Autodesk Inventor part; units mm, degrees
(part 2 of 2)
  spline S326 degree 2 poles (59.0858, 25.3317) (58.8361, 25.3317) (58.5495, 25.5905) (58.5495, 25.8217) knots 0 0 0 1 2 2 2
  spline S327 degree 2 poles (58.5495, 25.8217) (58.5495, 26.0482) (58.887, 26.3209) (59.1921, 26.3209) knots 0 0 0 1 2 2 2
  line L134 (59.1921, 26.3209) -> (59.3539, 26.3209)
  line L135 (65.4232, 23.2885) -> (65.4232, 23.307)
  spline S328 degree 2 poles (65.4232, 23.307) (65.3492, 23.0851) (64.9101, 22.7616) (64.397, 22.5952) (64.0919, 22.5952) knots 0 0 0 1 2 3 3 3
  spline S329 degree 2 poles (64.0919, 22.5952) (63.6851, 22.5952) (63.001, 22.9372) (62.5018, 23.5659) (62.2475, 24.4026) (62.2475, 24.8925) knots 0 0 0 1 2 3 4 4 4
  spline S330 degree 2 poles (62.2475, 24.8925) (62.2475, 25.9234) (63.2691, 27.0929) (64.1104, 27.0929) knots 0 0 0 1 2 2 2
  spline S331 degree 2 poles (64.1104, 27.0929) (64.5911, 27.0929) (65.2568, 26.76) (65.4232, 26.4503) knots 0 0 0 1 2 2 2
  line L136 (65.4232, 26.4503) -> (65.4232, 27.948)
  spline S332 degree 2 poles (65.4232, 27.948) (65.4232, 28.3039) (65.7283, 28.6922) (66.0149, 28.6922) knots 0 0 0 1 2 2 2
  spline S333 degree 2 poles (66.0149, 28.6922) (66.2922, 28.6922) (66.6019, 28.3317) (66.6019, 28.0035) knots 0 0 0 1 2 2 2
  line L137 (66.6019, 28.0035) -> (66.6019, 23.2885)
  spline S334 degree 2 poles (66.6019, 23.2885) (66.6019, 22.9511) (66.2737, 22.5952) (66.0149, 22.5952) knots 0 0 0 1 2 2 2
  spline S335 degree 2 poles (66.0149, 22.5952) (65.756, 22.5952) (65.4232, 22.9603) (65.4232, 23.2885) knots 0 0 0 1 2 2 2
  spline S336 degree 2 poles (63.4864, 24.8556) (63.4864, 24.4349) (63.7406, 23.8617) (64.1705, 23.5798) (64.4201, 23.5798) knots 0 0 0 1 2 3 3 3
  spline S337 degree 2 poles (64.4201, 23.5798) (64.679, 23.5798) (65.1042, 23.8479) (65.3631, 24.421) (65.3631, 24.8556) knots 0 0 0 1 2 3 3 3
  spline S338 degree 2 poles (65.3631, 24.8556) (65.3631, 25.2623) (65.1042, 25.8448) (64.6697, 26.1406) (64.4155, 26.1406) knots 0 0 0 1 2 3 3 3
  spline S339 degree 2 poles (64.4155, 26.1406) (64.1474, 26.1406) (63.7267, 25.8355) (63.4864, 25.2531) (63.4864, 24.8556) knots 0 0 0 1 2 3 3 3
  spline S340 degree 2 poles (68.4047, 22.5952) (68.1274, 22.5952) (67.7252, 22.9557) (67.7252, 23.2747) knots 0 0 0 1 2 2 2
  spline S341 degree 2 poles (67.7252, 23.2747) (67.7252, 23.5428) (68.1089, 23.9357) (68.3908, 23.9357) knots 0 0 0 1 2 2 2
  spline S342 degree 2 poles (68.3908, 23.9357) (68.6728, 23.9357) (69.0703, 23.5474) (69.0703, 23.2747) knots 0 0 0 1 2 2 2
  spline S343 degree 2 poles (69.0703, 23.2747) (69.0703, 22.9603) (68.6728, 22.5952) (68.4047, 22.5952) knots 0 0 0 1 2 2 2
  line L138 (71.3169, 26.4365) -> (71.3169, 26.3902)
  spline S344 degree 2 poles (71.3169, 26.3902) (71.4556, 26.7369) (72.1628, 27.1021) (72.6204, 27.1021) knots 0 0 0 1 2 2 2
  spline S345 degree 2 poles (72.6204, 27.1021) (73.0642, 27.1021) (73.7714, 26.7138) (73.9471, 26.3579) knots 0 0 0 1 2 2 2
  spline S346 degree 2 poles (73.9471, 26.3579) (74.058, 26.1499) (74.1227, 25.6737) (74.1227, 25.3178) knots 0 0 0 1 2 2 2
  line L139 (74.1227, 25.3178) -> (74.1227, 23.3301)
  spline S347 degree 2 poles (74.1227, 23.3301) (74.1227, 22.9742) (73.7853, 22.5952) (73.5126, 22.5952) knots 0 0 0 1 2 2 2
  spline S348 degree 2 poles (73.5126, 22.5952) (73.2352, 22.5952) (72.8932, 22.9835) (72.8932, 23.3301) knots 0 0 0 1 2 2 2
  line L140 (72.8932, 23.3301) -> (72.8932, 25.1098)
  spline S349 degree 2 poles (72.8932, 25.1098) (72.8932, 25.6183) (72.6297, 26.1175) (72.2414, 26.1175) knots 0 0 0 1 2 2 2
  spline S350 degree 2 poles (72.2414, 26.1175) (71.9825, 26.1175) (71.5572, 25.8078) (71.4417, 25.4981) knots 0 0 0 1 2 2 2
  spline S351 degree 2 poles (71.4417, 25.4981) (71.3816, 25.3132) (71.3816, 24.6707) knots 0 0 0 1 1 1
  line L141 (71.3816, 24.6707) -> (71.3816, 23.3301)
  spline S352 degree 2 poles (71.3816, 23.3301) (71.3816, 22.9696) (71.0349, 22.5952) (70.7576, 22.5952) knots 0 0 0 1 2 2 2
  spline S353 degree 2 poles (70.7576, 22.5952) (70.4895, 22.5952) (70.1474, 22.9835) (70.1474, 23.3301) knots 0 0 0 1 2 2 2
  line L142 (70.1474, 23.3301) -> (70.1474, 26.418)
  spline S354 degree 2 poles (70.1474, 26.418) (70.1474, 26.7508) (70.4571, 27.1021) (70.7252, 27.1021) knots 0 0 0 1 2 2 2
  spline S355 degree 2 poles (70.7252, 27.1021) (70.8916, 27.1021) (71.1597, 26.9449) (71.3169, 26.6398) (71.3169, 26.4365) knots 0 0 0 1 2 3 3 3
  line L143 (75.1258, 23.3301) -> (75.1258, 27.9619)
  spline S356 degree 2 poles (75.1258, 27.9619) (75.1258, 28.3132) (75.454, 28.6922) (75.736, 28.6922) knots 0 0 0 1 2 2 2
  spline S357 degree 2 poles (75.736, 28.6922) (76.018, 28.6922) (76.36, 28.3178) (76.36, 27.9619) knots 0 0 0 1 2 2 2
  line L144 (76.36, 27.9619) -> (76.36, 23.3301)
  spline S358 degree 2 poles (76.36, 23.3301) (76.36, 22.9696) (76.0133, 22.5952) (75.736, 22.5952) knots 0 0 0 1 2 2 2
  spline S359 degree 2 poles (75.736, 22.5952) (75.4633, 22.5952) (75.1258, 22.9835) (75.1258, 23.3301) knots 0 0 0 1 2 2 2
  line L145 (8.8947, 4.4889) -> (7.716, 4.4889)
  line L146 (7.716, 4.4889) -> (7.716, 5.9819)
  line L147 (7.716, 5.9819) -> (6.2183, 5.9819)
  line L148 (6.2183, 5.9819) -> (6.2183, 7.1699)
  line L149 (6.2183, 7.1699) -> (7.716, 7.1699)
  line L150 (7.716, 7.1699) -> (7.716, 8.6676)
  line L151 (7.716, 8.6676) -> (8.8947, 8.6676)
  line L152 (8.8947, 8.6676) -> (8.8947, 7.1699)
  line L153 (8.8947, 7.1699) -> (10.4016, 7.1699)
  line L154 (10.4016, 7.1699) -> (10.4016, 5.9819)
  line L155 (10.4016, 5.9819) -> (8.8947, 5.9819)
  line L156 (8.8947, 5.9819) -> (8.8947, 4.4889)
  spline S360 degree 2 poles (12.944, 7.2901) (13.2722, 7.2901) (13.7437, 7.6692) (13.7437, 8.0297) knots 0 0 0 1 2 2 2
  spline S361 degree 2 poles (13.7437, 8.0297) (13.7437, 8.2932) (13.3739, 8.6815) (13.0596, 8.6815) knots 0 0 0 1 2 2 2
  spline S362 degree 2 poles (13.0596, 8.6815) (12.8377, 8.6815) (12.5603, 8.5613) (12.4032, 8.3718) (12.2275, 7.9927) (12.1767, 7.8818) knots 0 0 0 1 2 3 4 4 4
  spline S363 degree 2 poles (12.1767, 7.8818) (12.1258, 7.7662) (11.8808, 7.6553) (11.7283, 7.6553) knots 0 0 0 1 2 2 2
  spline S364 degree 2 poles (11.7283, 7.6553) (11.5341, 7.6553) (11.2244, 7.9604) (11.2244, 8.2054) knots 0 0 0 1 2 2 2
  spline S365 degree 2 poles (11.2244, 8.2054) (11.2244, 8.4319) (11.4879, 8.908) (11.9871, 9.3333) (12.7175, 9.5921) (13.1659, 9.5921) knots 0 0 0 1 2 3 4 4 4
  spline S366 degree 2 poles (13.1659, 9.5921) (13.5588, 9.5921) (14.2152, 9.3749) (14.7052, 8.9588) (14.9548, 8.4134) (14.9548, 8.099) knots 0 0 0 1 2 3 4 4 4
  spline S367 degree 2 poles (14.9548, 8.099) (14.9548, 7.6876) (14.5942, 7.0913) (14.2984, 6.8926) knots 0 0 0 1 2 2 2
  spline S368 degree 2 poles (14.2984, 6.8926) (14.5711, 6.7816) (15.0103, 6.3379) (15.2321, 5.797) (15.2321, 5.4827) knots 0 0 0 1 2 3 3 3
  spline S369 degree 2 poles (15.2321, 5.4827) (15.2321, 5.1129) (14.9317, 4.4149) (14.3539, 3.8695) (13.5588, 3.5644) (13.0827, 3.5644) knots 0 0 0 1 2 3 4 4 4
  spline S370 degree 2 poles (13.0827, 3.5644) (12.5927, 3.5644) (11.8161, 3.9157) (11.3169, 4.4427) (11.058, 5.0112) (11.058, 5.2054) knots 0 0 0 1 2 3 4 4 4
  spline S371 degree 2 poles (11.058, 5.2054) (11.058, 5.4688) (11.4001, 5.7924) (11.6543, 5.7924) knots 0 0 0 1 2 2 2
  spline S372 degree 2 poles (11.6543, 5.7924) (11.7884, 5.7924) (12.0334, 5.6306) (12.0796, 5.4873) knots 0 0 0 1 2 2 2
  spline S373 degree 2 poles (12.0796, 5.4873) (12.2737, 4.9881) (12.7036, 4.4981) (13.0919, 4.4981) knots 0 0 0 1 2 2 2
  spline S374 degree 2 poles (13.0919, 4.4981) (13.3138, 4.4981) (13.7206, 4.7154) (13.9933, 5.1499) (13.9933, 5.4365) knots 0 0 0 1 2 3 3 3
  spline S375 degree 2 poles (13.9933, 5.4365) (13.9933, 5.8618) (13.5357, 6.3333) (13.1289, 6.3333) knots 0 0 0 1 2 2 2
  spline S376 degree 2 poles (13.1289, 6.3333) (13.0596, 6.3333) (12.7314, 6.3009) (12.6759, 6.3009) knots 0 0 0 1 2 2 2
  spline S377 degree 2 poles (12.6759, 6.3009) (12.4263, 6.3009) (12.1397, 6.5598) (12.1397, 6.7909) knots 0 0 0 1 2 2 2
  spline S378 degree 2 poles (12.1397, 6.7909) (12.1397, 7.0174) (12.4771, 7.2901) (12.7822, 7.2901) knots 0 0 0 1 2 2 2
  line L157 (12.7822, 7.2901) -> (12.944, 7.2901)
  line L158 (17.7976, 4.2809) -> (17.7976, 7.7616)
  spline S379 degree 2 poles (17.7976, 7.7616) (16.9147, 6.9989) (16.5403, 6.9989) knots 0 0 0 1 1 1
  spline S380 degree 2 poles (16.5403, 6.9989) (16.3415, 6.9989) (16.0411, 7.3086) (16.0411, 7.5166) knots 0 0 0 1 2 2 2
  spline S381 degree 2 poles (16.0411, 7.5166) (16.0411, 7.757) (16.323, 7.9696) (16.6559, 8.1222) knots 0 0 0 1 2 2 2
  spline S382 degree 2 poles (16.6559, 8.1222) (17.1135, 8.3394) (17.6636, 8.8202) (18.0981, 9.4211) (18.2645, 9.6014) (18.4864, 9.6014) knots 0 0 0 1 2 3 4 4 4
  spline S383 degree 2 poles (18.4864, 9.6014) (18.736, 9.6014) (19.0272, 9.2269) (19.0272, 8.9219) knots 0 0 0 1 2 2 2
  line L159 (19.0272, 8.9219) -> (19.0272, 4.4334)
  spline S384 degree 2 poles (19.0272, 4.4334) (19.0272, 3.5644) (18.4078, 3.5644) knots 0 0 0 1 1 1
  spline S385 degree 2 poles (18.4078, 3.5644) (18.1304, 3.5644) (17.7976, 3.9342) (17.7976, 4.2809) knots 0 0 0 1 2 2 2
  spline S386 degree 2 poles (20.9039, 5.8202) (20.9039, 6.4211) (21.1119, 7.4658) (21.528, 8.4688) (21.8423, 8.9819) knots 0 0 0 1 2 3 3 3
  spline S387 degree 2 poles (21.8423, 8.9819) (22.0272, 9.2917) (22.2999, 9.5829) (22.5588, 9.6615) (22.7483, 9.6615) knots 0 0 0 1 2 3 3 3
  spline S388 degree 2 poles (22.7483, 9.6615) (23.021, 9.6615) (23.021, 9.4766) knots 0 0 0 1 1 1
  spline S389 degree 2 poles (23.021, 9.4766) (23.021, 9.4257) (22.6512, 8.6214) (22.3415, 7.7893) (22.0734, 6.5274) (22.0734, 5.8202) knots 0 0 0 1 2 3 4 4 4
  spline S390 degree 2 poles (22.0734, 5.8202) (22.0734, 5.1175) (22.3369, 3.8787) (22.6744, 2.9588) (23.021, 2.2146) (23.021, 2.1684) knots 0 0 0 1 2 3 4 4 4
  spline S391 degree 2 poles (23.021, 2.1684) (23.021, 1.9789) (22.7483, 1.9789) knots 0 0 0 1 1 1
  spline S392 degree 2 poles (22.7483, 1.9789) (22.5495, 1.9789) (22.2953, 2.0621) (22.0318, 2.3625) (21.8608, 2.6353) knots 0 0 0 1 2 3 3 3
  spline S393 degree 2 poles (21.8608, 2.6353) (21.528, 3.19) (21.1166, 4.1653) (20.9039, 5.21) (20.9039, 5.8202) knots 0 0 0 1 2 3 3 3
  spline S394 degree 2 poles (27.8515, 6.5598) (27.8515, 5.9126) (27.6898, 4.9696) (27.4725, 4.5767) knots 0 0 0 1 2 2 2
  spline S395 degree 2 poles (27.4725, 4.5767) (27.1952, 4.096) (26.3123, 3.5736) (25.7714, 3.5736) knots 0 0 0 1 2 2 2
  spline S396 degree 2 poles (25.7714, 3.5736) (25.1474, 3.5736) (24.1628, 4.2762) (23.9178, 4.8772) knots 0 0 0 1 2 2 2
  spline S397 degree 2 poles (23.9178, 4.8772) (23.7884, 5.2331) (23.6728, 6.0235) (23.6728, 6.495) knots 0 0 0 1 2 2 2
  spline S398 degree 2 poles (23.6728, 6.495) (23.6728, 7.096) (23.7976, 8.0482) (23.9455, 8.4272) knots 0 0 0 1 2 2 2
  spline S399 degree 2 poles (23.9455, 8.4272) (24.1767, 8.9866) (25.1012, 9.606) (25.7391, 9.606) knots 0 0 0 1 2 2 2
  spline S400 degree 2 poles (25.7391, 9.606) (26.1551, 9.606) (26.8485, 9.3286) (27.3708, 8.8017) (27.5465, 8.4226) knots 0 0 0 1 2 3 3 3
  spline S401 degree 2 poles (27.5465, 8.4226) (27.8515, 7.757) (27.8515, 6.5598) knots 0 0 0 1 1 1
  spline S402 degree 2 poles (26.6127, 6.6383) (26.6127, 7.3456) (26.4463, 8.2285) (26.0765, 8.6491) (25.7529, 8.6491) knots 0 0 0 1 2 3 3 3
  spline S403 degree 2 poles (25.7529, 8.6491) (25.2953, 8.6491) (24.9163, 7.6784) (24.9163, 6.606) knots 0 0 0 1 2 2 2
  spline S404 degree 2 poles (24.9163, 6.606) (24.9163, 5.871) (25.0827, 4.965) (25.4525, 4.5305) (25.7622, 4.5305) knots 0 0 0 1 2 3 3 3
  spline S405 degree 2 poles (25.7622, 4.5305) (26.0811, 4.5305) (26.4509, 4.9835) (26.6127, 5.8987) (26.6127, 6.6383) knots 0 0 0 1 2 3 3 3
  spline S406 degree 2 poles (30.6759, 5.8202) (30.6759, 4.9465) (30.209, 3.4442) (29.7375, 2.6676) knots 0 0 0 1 2 2 2
  spline S407 degree 2 poles (29.7375, 2.6676) (29.4694, 2.2239) (29.1274, 1.9789) (28.8361, 1.9789) knots 0 0 0 1 2 2 2
  spline S408 degree 2 poles (28.8361, 1.9789) (28.5588, 1.9789) (28.5588, 2.1684) knots 0 0 0 1 1 1
  spline S409 degree 2 poles (28.5588, 2.1684) (28.5588, 2.2192) (28.8962, 2.9172) (29.2475, 3.8556) (29.5064, 5.1222) (29.5064, 5.8202) knots 0 0 0 1 2 3 4 4 4
  spline S410 degree 2 poles (29.5064, 5.8202) (29.5064, 6.5182) (29.2429, 7.7893) (28.8962, 8.7185) (28.5588, 9.4257) (28.5588, 9.4766) knots 0 0 0 1 2 3 4 4 4
  spline S411 degree 2 poles (28.5588, 9.4766) (28.5588, 9.6615) (28.8361, 9.6615) knots 0 0 0 1 1 1
  spline S412 degree 2 poles (28.8361, 9.6615) (29.1366, 9.6615) (29.474, 9.4257) (29.7514, 8.908) knots 0 0 0 1 2 2 2
  spline S413 degree 2 poles (29.7514, 8.908) (29.9733, 8.589) (30.32, 7.8402) (30.5557, 7.0867) (30.6759, 6.2639) (30.6759, 5.8202) knots 0 0 0 1 2 3 4 4 4
  spline S414 degree 2 poles (32.6867, 6.9342) (32.8115, 7.23) (33.4725, 7.5536) (33.8839, 7.5536) knots 0 0 0 1 2 2 2
  spline S415 degree 2 poles (33.8839, 7.5536) (34.2722, 7.5536) (34.9378, 7.2578) (35.4324, 6.7215) (35.7005, 6.0004) (35.7005, 5.6075) knots 0 0 0 1 2 3 4 4 4
  spline S416 degree 2 poles (35.7005, 5.6075) (35.7005, 5.0343) (35.1736, 4.0913) (34.2306, 3.5644) (33.6343, 3.5644) knots 0 0 0 1 2 3 3 3
  spline S417 degree 2 poles (33.6343, 3.5644) (32.9502, 3.5644) (31.9563, 4.2346) (31.434, 5.5289) (31.434, 6.4581) knots 0 0 0 1 2 3 3 3
  spline S418 degree 2 poles (31.434, 6.4581) (31.434, 7.2069) (31.7437, 8.3995) (32.3354, 9.19) (33.1905, 9.6014) (33.7314, 9.6014) knots 0 0 0 1 2 3 4 4 4
  spline S419 degree 2 poles (33.7314, 9.6014) (34.2491, 9.6014) (35.0534, 9.19) (35.4648, 8.5752) (35.4648, 8.2839) knots 0 0 0 1 2 3 3 3
  spline S420 degree 2 poles (35.4648, 8.2839) (35.4648, 8.0944) (35.1736, 7.7801) (34.9517, 7.7801) knots 0 0 0 1 2 2 2
  spline S421 degree 2 poles (34.9517, 7.7801) (34.7576, 7.7801) (34.434, 8.0158) (34.3554, 8.2608) knots 0 0 0 1 2 2 2
  spline S422 degree 2 poles (34.3554, 8.2608) (34.2814, 8.4365) (33.9301, 8.6907) (33.699, 8.6907) knots 0 0 0 1 2 2 2
  spline S423 degree 2 poles (33.699, 8.6907) (33.5141, 8.6907) (33.1351, 8.4688) (33.0056, 8.2839) knots 0 0 0 1 2 2 2
  spline S424 degree 2 poles (33.0056, 8.2839) (32.7329, 7.8864) (32.6867, 6.9342) knots 0 0 0 1 1 1
  spline S425 degree 2 poles (33.662, 4.4981) (34.0133, 4.4981) (34.4895, 5.0898) (34.4895, 5.589) knots 0 0 0 1 2 2 2
  spline S426 degree 2 poles (34.4895, 5.589) (34.4895, 5.9265) (34.2629, 6.4026) (33.8793, 6.6476) (33.6528, 6.6476) knots 0 0 0 1 2 3 3 3
  spline S427 degree 2 poles (33.6528, 6.6476) (33.4309, 6.6476) (33.0287, 6.4118) (32.7791, 5.9635) (32.7791, 5.6537) knots 0 0 0 1 2 3 3 3
  spline S428 degree 2 poles (32.7791, 5.6537) (32.7791, 5.1499) (33.2876, 4.4981) (33.662, 4.4981) knots 0 0 0 1 2 2 2
  spline S429 degree 2 poles (38.2106, 7.2901) (38.5388, 7.2901) (39.0103, 7.6692) (39.0103, 8.0297) knots 0 0 0 1 2 2 2
  spline S430 degree 2 poles (39.0103, 8.0297) (39.0103, 8.2932) (38.6405, 8.6815) (38.3261, 8.6815) knots 0 0 0 1 2 2 2
  spline S431 degree 2 poles (38.3261, 8.6815) (38.1042, 8.6815) (37.8269, 8.5613) (37.6697, 8.3718) (37.4941, 7.9927) (37.4432, 7.8818) knots 0 0 0 1 2 3 4 4 4
  spline S432 degree 2 poles (37.4432, 7.8818) (37.3924, 7.7662) (37.1474, 7.6553) (36.9948, 7.6553) knots 0 0 0 1 2 2 2
  spline S433 degree 2 poles (36.9948, 7.6553) (36.8007, 7.6553) (36.491, 7.9604) (36.491, 8.2054) knots 0 0 0 1 2 2 2
  spline S434 degree 2 poles (36.491, 8.2054) (36.491, 8.4319) (36.7545, 8.908) (37.2537, 9.3333) (37.9841, 9.5921) (38.4324, 9.5921) knots 0 0 0 1 2 3 4 4 4
  spline S435 degree 2 poles (38.4324, 9.5921) (38.8254, 9.5921) (39.4817, 9.3749) (39.9717, 8.9588) (40.2213, 8.4134) (40.2213, 8.099) knots 0 0 0 1 2 3 4 4 4
  spline S436 degree 2 poles (40.2213, 8.099) (40.2213, 7.6876) (39.8608, 7.0913) (39.565, 6.8926) knots 0 0 0 1 2 2 2
  spline S437 degree 2 poles (39.565, 6.8926) (39.8377, 6.7816) (40.2768, 6.3379) (40.4987, 5.797) (40.4987, 5.4827) knots 0 0 0 1 2 3 3 3
  spline S438 degree 2 poles (40.4987, 5.4827) (40.4987, 5.1129) (40.1982, 4.4149) (39.6204, 3.8695) (38.8254, 3.5644) (38.3492, 3.5644) knots 0 0 0 1 2 3 4 4 4
  spline S439 degree 2 poles (38.3492, 3.5644) (37.8593, 3.5644) (37.0827, 3.9157) (36.5834, 4.4427) (36.3246, 5.0112) (36.3246, 5.2054) knots 0 0 0 1 2 3 4 4 4
  spline S440 degree 2 poles (36.3246, 5.2054) (36.3246, 5.4688) (36.6666, 5.7924) (36.9209, 5.7924) knots 0 0 0 1 2 2 2
  spline S441 degree 2 poles (36.9209, 5.7924) (37.0549, 5.7924) (37.2999, 5.6306) (37.3462, 5.4873) knots 0 0 0 1 2 2 2
  spline S442 degree 2 poles (37.3462, 5.4873) (37.5403, 4.9881) (37.9702, 4.4981) (38.3585, 4.4981) knots 0 0 0 1 2 2 2
  spline S443 degree 2 poles (38.3585, 4.4981) (38.5804, 4.4981) (38.9871, 4.7154) (39.2599, 5.1499) (39.2599, 5.4365) knots 0 0 0 1 2 3 3 3
  spline S444 degree 2 poles (39.2599, 5.4365) (39.2599, 5.8618) (38.8022, 6.3333) (38.3955, 6.3333) knots 0 0 0 1 2 2 2
  spline S445 degree 2 poles (38.3955, 6.3333) (38.3261, 6.3333) (37.9979, 6.3009) (37.9425, 6.3009) knots 0 0 0 1 2 2 2
  spline S446 degree 2 poles (37.9425, 6.3009) (37.6928, 6.3009) (37.4062, 6.5598) (37.4062, 6.7909) knots 0 0 0 1 2 2 2
  spline S447 degree 2 poles (37.4062, 6.7909) (37.4062, 7.0174) (37.7437, 7.2901) (38.0488, 7.2901) knots 0 0 0 1 2 2 2
  line L160 (38.0488, 7.2901) -> (38.2106, 7.2901)
  line L161 (43.0642, 4.2809) -> (43.0642, 7.7616)
  spline S448 degree 2 poles (43.0642, 7.7616) (42.1813, 6.9989) (41.8069, 6.9989) knots 0 0 0 1 1 1
  spline S449 degree 2 poles (41.8069, 6.9989) (41.6081, 6.9989) (41.3076, 7.3086) (41.3076, 7.5166) knots 0 0 0 1 2 2 2
  spline S450 degree 2 poles (41.3076, 7.5166) (41.3076, 7.757) (41.5896, 7.9696) (41.9224, 8.1222) knots 0 0 0 1 2 2 2
  spline S451 degree 2 poles (41.9224, 8.1222) (42.3801, 8.3394) (42.9301, 8.8202) (43.3646, 9.4211) (43.5311, 9.6014) (43.7529, 9.6014) knots 0 0 0 1 2 3 4 4 4
  spline S452 degree 2 poles (43.7529, 9.6014) (44.0025, 9.6014) (44.2938, 9.2269) (44.2938, 8.9219) knots 0 0 0 1 2 2 2
  line L162 (44.2938, 8.9219) -> (44.2938, 4.4334)
  spline S453 degree 2 poles (44.2938, 4.4334) (44.2938, 3.5644) (43.6744, 3.5644) knots 0 0 0 1 1 1
  spline S454 degree 2 poles (43.6744, 3.5644) (43.397, 3.5644) (43.0642, 3.9342) (43.0642, 4.2809) knots 0 0 0 1 2 2 2
  line L163 (47.622, 4.7477) -> (49.5865, 4.7477)
  spline S455 degree 2 poles (49.5865, 4.7477) (49.9193, 4.7477) (50.2938, 4.4565) (50.2938, 4.2023) knots 0 0 0 1 2 2 2
  spline S456 degree 2 poles (50.2938, 4.2023) (50.2938, 3.9758) (49.9933, 3.6615) (49.6975, 3.6615) knots 0 0 0 1 2 2 2
  line L164 (49.6975, 3.6615) -> (46.8176, 3.6615)
  spline S457 degree 2 poles (46.8176, 3.6615) (46.4895, 3.6615) (46.1104, 4.0359) (46.1104, 4.2901) knots 0 0 0 1 2 2 2
  spline S458 degree 2 poles (46.1104, 4.2901) (46.1104, 4.4473) (46.3323, 4.9373) (46.5172, 5.1129) knots 0 0 0 1 2 2 2
  spline S459 degree 2 poles (46.5172, 5.1129) (46.9933, 5.626) (47.8346, 6.4026) (48.0334, 6.5366) knots 0 0 0 1 2 2 2
  spline S460 degree 2 poles (48.0334, 6.5366) (48.3338, 6.7493) (48.7452, 7.1884) (48.9579, 7.6507) (48.9579, 7.8633) knots 0 0 0 1 2 3 3 3
  spline S461 degree 2 poles (48.9579, 7.8633) (48.9579, 8.0898) (48.7406, 8.4457) (48.3662, 8.6445) (48.1489, 8.6445) knots 0 0 0 1 2 3 3 3
  spline S462 degree 2 poles (48.1489, 8.6445) (47.6774, 8.6445) (47.4093, 8.2331) knots 0 0 0 1 1 1
  spline S463 degree 2 poles (47.4093, 8.2331) (47.377, 8.1823) (47.1921, 7.6507) (46.9286, 7.3271) (46.6651, 7.3271) knots 0 0 0 1 2 3 3 3
  spline S464 degree 2 poles (46.6651, 7.3271) (46.434, 7.3271) (46.1289, 7.6322) (46.1289, 7.891) knots 0 0 0 1 2 2 2
  spline S465 degree 2 poles (46.1289, 7.891) (46.1289, 8.1823) (46.3785, 8.7924) (46.8824, 9.2963) (47.6589, 9.6014) (48.172, 9.6014) knots 0 0 0 1 2 3 4 4 4
  spline S466 degree 2 poles (48.172, 9.6014) (48.7868, 9.6014) (49.226, 9.4072) knots 0 0 0 1 1 1
  spline S467 degree 2 poles (49.226, 9.4072) (49.5172, 9.2732) (49.9563, 8.8109) (50.1967, 8.2054) (50.1967, 7.8864) knots 0 0 0 1 2 3 3 3
  spline S468 degree 2 poles (50.1967, 7.8864) (50.1967, 7.3779) (49.6975, 6.5505) (49.1797, 6.0883) (48.0103, 5.1314) (47.7976, 4.8725) knots 0 0 0 1 2 3 4 4 4
  spline S469 degree 2 poles (47.7976, 4.8725) (47.7052, 4.7709) (47.622, 4.7477) knots 0 0 0 1 1 1
  line L165 (51.87, 9.5089) -> (54.4771, 9.5089)
  spline S470 degree 2 poles (54.4771, 9.5089) (54.8793, 9.5089) (55.2722, 9.2362) (55.2722, 8.9265) knots 0 0 0 1 2 2 2
  spline S471 degree 2 poles (55.2722, 8.9265) (55.2722, 8.7323) (54.8469, 8.1545) (54.3569, 7.5212) (53.8254, 6.5598) (53.6127, 5.9311) knots 0 0 0 1 2 3 4 4 4
  spline S472 degree 2 poles (53.6127, 5.9311) (53.511, 5.5613) (53.4371, 5.1776) (53.3446, 4.5259) (53.3076, 4.341) knots 0 0 0 1 2 3 3 3
  spline S473 degree 2 poles (53.3076, 4.341) (53.2198, 3.9157) (52.8777, 3.5644) (52.5911, 3.5644) knots 0 0 0 1 2 2 2
  spline S474 degree 2 poles (52.5911, 3.5644) (52.3138, 3.5644) (51.981, 3.948) (51.981, 4.304) knots 0 0 0 1 2 2 2
  spline S475 degree 2 poles (51.981, 4.304) (51.981, 4.5675) (52.1936, 5.4365) (52.6744, 6.6476) (53.4001, 7.928) (53.8808, 8.4272) knots 0 0 0 1 2 3 4 4 4
  line L166 (53.8808, 8.4272) -> (51.87, 8.4272)
  spline S476 degree 2 poles (51.87, 8.4272) (51.5095, 8.4272) (51.1304, 8.7046) (51.1304, 9.0051) knots 0 0 0 1 2 2 2
  spline S477 degree 2 poles (51.1304, 9.0051) (51.1304, 9.324) (51.5372, 9.5089) (51.87, 9.5089) knots 0 0 0 1 2 2 2
  line L167 (57.6666, 4.2809) -> (57.6666, 7.7616)
  spline S478 degree 2 poles (57.6666, 7.7616) (56.7838, 6.9989) (56.4093, 6.9989) knots 0 0 0 1 1 1
  spline S479 degree 2 poles (56.4093, 6.9989) (56.2106, 6.9989) (55.9101, 7.3086) (55.9101, 7.5166) knots 0 0 0 1 2 2 2
  spline S480 degree 2 poles (55.9101, 7.5166) (55.9101, 7.757) (56.1921, 7.9696) (56.5249, 8.1222) knots 0 0 0 1 2 2 2
  spline S481 degree 2 poles (56.5249, 8.1222) (56.9825, 8.3394) (57.5326, 8.8202) (57.9671, 9.4211) (58.1335, 9.6014) (58.3554, 9.6014) knots 0 0 0 1 2 3 4 4 4
  spline S482 degree 2 poles (58.3554, 9.6014) (58.605, 9.6014) (58.8962, 9.2269) (58.8962, 8.9219) knots 0 0 0 1 2 2 2
  line L168 (58.8962, 8.9219) -> (58.8962, 4.4334)
  spline S483 degree 2 poles (58.8962, 4.4334) (58.8962, 3.5644) (58.2768, 3.5644) knots 0 0 0 1 1 1
  spline S484 degree 2 poles (58.2768, 3.5644) (57.9995, 3.5644) (57.6666, 3.9342) (57.6666, 4.2809) knots 0 0 0 1 2 2 2
  line L169 (61.605, 9.5089) -> (64.2121, 9.5089)
  spline S485 degree 2 poles (64.2121, 9.5089) (64.6143, 9.5089) (65.0072, 9.2362) (65.0072, 8.9265) knots 0 0 0 1 2 2 2
  spline S486 degree 2 poles (65.0072, 8.9265) (65.0072, 8.7323) (64.5819, 8.1545) (64.0919, 7.5212) (63.5603, 6.5598) (63.3477, 5.9311) knots 0 0 0 1 2 3 4 4 4
  spline S487 degree 2 poles (63.3477, 5.9311) (63.246, 5.5613) (63.172, 5.1776) (63.0796, 4.5259) (63.0426, 4.341) knots 0 0 0 1 2 3 3 3
  spline S488 degree 2 poles (63.0426, 4.341) (62.9548, 3.9157) (62.6127, 3.5644) (62.3261, 3.5644) knots 0 0 0 1 2 2 2
  spline S489 degree 2 poles (62.3261, 3.5644) (62.0488, 3.5644) (61.716, 3.948) (61.716, 4.304) knots 0 0 0 1 2 2 2
  spline S490 degree 2 poles (61.716, 4.304) (61.716, 4.5675) (61.9286, 5.4365) (62.4093, 6.6476) (63.1351, 7.928) (63.6158, 8.4272) knots 0 0 0 1 2 3 4 4 4
  line L170 (63.6158, 8.4272) -> (61.605, 8.4272)
  spline S491 degree 2 poles (61.605, 8.4272) (61.2445, 8.4272) (60.8654, 8.7046) (60.8654, 9.0051) knots 0 0 0 1 2 2 2
  spline S492 degree 2 poles (60.8654, 9.0051) (60.8654, 9.324) (61.2722, 9.5089) (61.605, 9.5089) knots 0 0 0 1 2 2 2
  line L171 (67.4016, 4.2809) -> (67.4016, 7.7616)
  spline S493 degree 2 poles (67.4016, 7.7616) (66.5187, 6.9989) (66.1443, 6.9989) knots 0 0 0 1 1 1
  spline S494 degree 2 poles (66.1443, 6.9989) (65.9455, 6.9989) (65.6451, 7.3086) (65.6451, 7.5166) knots 0 0 0 1 2 2 2
  spline S495 degree 2 poles (65.6451, 7.5166) (65.6451, 7.757) (65.927, 7.9696) (66.2599, 8.1222) knots 0 0 0 1 2 2 2
  spline S496 degree 2 poles (66.2599, 8.1222) (66.7175, 8.3394) (67.2676, 8.8202) (67.7021, 9.4211) (67.8685, 9.6014) (68.0904, 9.6014) knots 0 0 0 1 2 3 4 4 4
  spline S497 degree 2 poles (68.0904, 9.6014) (68.34, 9.6014) (68.6312, 9.2269) (68.6312, 8.9219) knots 0 0 0 1 2 2 2
  line L172 (68.6312, 8.9219) -> (68.6312, 4.4334)
  spline S498 degree 2 poles (68.6312, 4.4334) (68.6312, 3.5644) (68.0118, 3.5644) knots 0 0 0 1 1 1
  spline S499 degree 2 poles (68.0118, 3.5644) (67.7344, 3.5644) (67.4016, 3.9342) (67.4016, 4.2809) knots 0 0 0 1 2 2 2
  line L173 (71.34, 9.5089) -> (73.9471, 9.5089)
  spline S500 degree 2 poles (73.9471, 9.5089) (74.3492, 9.5089) (74.7421, 9.2362) (74.7421, 8.9265) knots 0 0 0 1 2 2 2
  spline S501 degree 2 poles (74.7421, 8.9265) (74.7421, 8.7323) (74.3169, 8.1545) (73.8269, 7.5212) (73.2953, 6.5598) (73.0827, 5.9311) knots 0 0 0 1 2 3 4 4 4
  spline S502 degree 2 poles (73.0827, 5.9311) (72.981, 5.5613) (72.907, 5.1776) (72.8146, 4.5259) (72.7776, 4.341) knots 0 0 0 1 2 3 3 3
  spline S503 degree 2 poles (72.7776, 4.341) (72.6898, 3.9157) (72.3477, 3.5644) (72.0611, 3.5644) knots 0 0 0 1 2 2 2
  spline S504 degree 2 poles (72.0611, 3.5644) (71.7838, 3.5644) (71.4509, 3.948) (71.4509, 4.304) knots 0 0 0 1 2 2 2
  spline S505 degree 2 poles (71.4509, 4.304) (71.4509, 4.5675) (71.6636, 5.4365) (72.1443, 6.6476) (72.87, 7.928) (73.3508, 8.4272) knots 0 0 0 1 2 3 4 4 4
  line L174 (73.3508, 8.4272) -> (71.34, 8.4272)
  spline S506 degree 2 poles (71.34, 8.4272) (70.9794, 8.4272) (70.6004, 8.7046) (70.6004, 9.0051) knots 0 0 0 1 2 2 2
  spline S507 degree 2 poles (70.6004, 9.0051) (70.6004, 9.324) (71.0072, 9.5089) (71.34, 9.5089) knots 0 0 0 1 2 2 2
  dimension "d0" = 85
  dimension "d1" = 50
  constraints: 8 end point, 2 parallel, 1 horizontal, 1 perpendicular, 2 other
  measures "d0" distance of L2.end L1.end
  measures "d1" distance of L2.end L0.start
extrude "Extrusion1" add sketch "Sketch1" along normal blind 0.6
body "Solid1"
